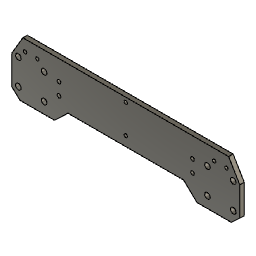
lcd_cover_prusa (Autodesk Fusion 360 archive; units mm, degrees)
design "front_plate"
Autodesk Fusion 360 part; units mm, degrees
sketch "MK3-front-plate" plane through (0, 0, 0) normal (0, 1, 0) x (1, 0, 0)
  line L0 (-64, 0) -> (-95, 0)
  line L1 (-95, 0) -> (-102.5, -7)
  line L2 (-102.5, -7) -> (-102.5, -33)
  line L3 (-102.5, -33) -> (-92.5, -50)
  line L4 (-92.5, -50) -> (92.5, -50)
  line L5 (102.5, -33) -> (102.5, -7)
  line L6 (64, 0) -> (52, -11.5)
  line L7 (102.5, -7) -> (95, 0)
  line L8 (-52, -11.5) -> (-64, 0)
  line L9 (95, 0) -> (64, 0)
  line L10 (52, -11.5) -> (-52, -11.5)
  line L11 (92.5, -50) -> (102.5, -33)
  line L12 (-64, 0) -> (64, 0) construction
  line L13 (-73.4, 0) -> (-73.4, -50) construction
  line L14 (-96.6, 0) -> (-96.6, -50) construction
  circle A0 centre (-73.4, -9.9) radius 2.5
  circle A1 centre (-96.6, -9.9) radius 2.5
  circle A2 centre (-73.4, -33.1) radius 2.5
  circle A3 centre (-96.6, -33.1) radius 2.5
  line L15 (-96.6, -40) -> (-73.4, -40) construction
  circle A4 centre (-90.5, -40) radius 1.5
  circle A5 centre (-79.5, -40) radius 1.5
  circle A6 centre (0, -46) radius 1.5
  line L16 (0, 0) -> (0, -50) construction
  circle A7 centre (0, -20) radius 1.5
  line L17 (-60, -21) -> (-60, -32) construction
  circle A8 centre (-60, -21) radius 1.65
  circle A9 centre (-60, -32) radius 1.65
  circle A10 centre (60, -32) radius 1.65
  circle A11 centre (60, -21) radius 1.65
  circle A12 centre (73.4, -9.9) radius 2.5
  circle A13 centre (96.6, -9.9) radius 2.5
  circle A14 centre (96.6, -33.1) radius 2.5
  circle A15 centre (73.4, -33.1) radius 2.5
  circle A16 centre (79.5, -40) radius 1.5
  circle A17 centre (90.5, -40) radius 1.5
  line L18 (0, -33.1) -> (-102.5, -33.1) construction
  line L19 (-102.5, -9.9) -> (0, -9.9) construction
  dimension "d3" = 50
  dimension "d4" = 205
  dimension "d5" = 7.5
  dimension "d12" = 10
  dimension "d16" = 17
  dimension "d26" = 5
  dimension "d27" = 5
  dimension "d28" = 5
  dimension "d29" = 5
  dimension "d37" = 3
  dimension "d40" = 3
  dimension "d46" = 4
  dimension "d48" = 3
  dimension "d49" = 3
  dimension "d50" = 10
  dimension "d51" = 16.9
  dimension "d52" = 3.3
  dimension "d53" = 3.3
  dimension "d54" = 18
  dimension "d56" = 42.5
  dimension "d57" = 5.9
  dimension "d58" = 29.1
  dimension "d59" = 40.1
  dimension "d60" = 102.5
  dimension "d61" = 43
  dimension "d62" = 29
  dimension "d63" = 12
  dimension "d64" = 23
  dimension "d65" = 50.5
  dimension "d66" = 12
  dimension "d67" = 38.5
  dimension "d68" = 30
  constraint parallel L9 L12
  constraint midpoint L16.start L12
  constraint coincident L0 L13.start
  constraint coincident L4 L13.end
  constraint perpendicular L4 L13
  constraint coincident L0 L14.start
  constraint coincident L4 L14.end
  constraint perpendicular L4 L14
  constraint coincident L2 L19.start
  constraint coincident L2 L18.end
  constraint coincident L13 A0.centre
  constraint coincident A0.centre L19
  constraint coincident L14 A1.centre
  constraint coincident A1.centre L19
  constraint coincident L13 A2.centre
  constraint coincident L14 A3.centre
  constraint coincident L14 L15.start
  constraint coincident L13 L15.end
  constraint perpendicular L13 L15
  constraint coincident L15 A4.centre
  constraint coincident L15 A5.centre
  constraint coincident L16.start origin
  constraint midpoint L4 L16.end
  constraint coincident L16 A7.centre
  constraint coincident A6.centre L16
  constraint symmetric L3 L11 L16
  constraint symmetric L1 L7 L16
  constraint coincident L17.start A8.centre
  constraint coincident L17.end A9.centre
  constraint vertical L17
  constraint symmetric L16 A8 A11
  constraint symmetric L16 A9 A10
  constraint symmetric L2 L5 L16
  constraint symmetric A0 L16 A12
  constraint symmetric A1 L16 A13
  constraint symmetric A2 L16 A15
  constraint symmetric A3 L16 A14
  constraint symmetric A4 L16 A17
  constraint symmetric A5 L16 A16
  constraint symmetric L6 L8 L16
  constraint coincident L16 L18.start
  constraint coincident L16 L19.end
  constraint perpendicular L16 L18
  constraint perpendicular L16 L19
  constraint coincident A2.centre L18
  constraint coincident A3.centre L18
  measures "d3" distance of L0 L4
  measures "d4" distance of L2 L5
  measures "d5" distance of L0.end L2
  measures "d12" horizontal distance of L2.end L3.end
  measures "d16" vertical distance of L2.end L3.end
  measures "d26" diameter of A0
  measures "d27" diameter of A1
  measures "d28" diameter of A2
  measures "d29" diameter of A3
  measures "d37" diameter of A4
  measures "d40" diameter of A5
  measures "d46" distance of L4 A6.centre
  measures "d48" diameter of A7
  measures "d49" diameter of A6
  measures "d50" distance of L4 L15.end
  measures "d51" vertical distance of L3.end L18.end
  measures "d52" diameter of A9
  measures "d53" diameter of A8
  measures "d54" distance of L4 L17.end
  measures "d56" distance of L2 L17.end
  measures "d57" horizontal distance of L1.end L14.start
  measures "d58" horizontal distance of L1.end L13.start
  measures "d59" vertical distance of L3.end L19.start
  measures "d60" horizontal distance of L16.start L1.end
  measures "d61" vertical distance of L1.end L3.end
  measures "d62" distance of L4 L17.start
  measures "d63" horizontal distance of L18.end A4.centre
  measures "d64" horizontal distance of L18.end A5.centre
  measures "d65" horizontal distance of L1.end L8.start
  measures "d66" horizontal distance of L0.start L8.start
  measures "d67" distance of L4 L10
  measures "d68" distance of L4 A7.centre
extrude "Extrude1" add sketch "MK3-front-plate" along normal blind 4
equation "d38 = ( ( 23.2 - 11 ) / 2 ) * 1 mm"
equation "d43 = ( ( 23.2 - 11 ) / 2 ) * 1 mm"

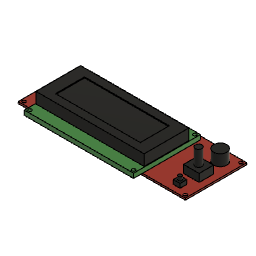
design "lcd"
Autodesk Fusion 360 part; units mm, degrees
sketch "Sketch1" plane through (0, 0, 0) normal (0, 0, 1) x (1, 0, 0)
  line L0 (150, 55) -> (150, 0)
  line L1 (150, 0) -> (0, 0)
  line L2 (0, 55) -> (150, 55)
  line L3 (68.5, 32.5) -> (66.3, 32.5) construction
  line L4 (66.3, 32.5) -> (66.3, 23.5)
  line L5 (0, 0) -> (0, 55)
  line L6 (89, 32.5) -> (89, 23.5)
  line L7 (45.8, 32.5) -> (66.3, 32.5)
  line L8 (89, 23.5) -> (68.5, 23.5)
  line L9 (66.3, 23.5) -> (45.8, 23.5)
  line L10 (68.5, 32.5) -> (89, 32.5)
  line L11 (68.5, 23.5) -> (68.5, 32.5)
  line L12 (45.8, 23.5) -> (45.8, 32.5)
  circle A0 centre (2.6, 2.6) radius 1.5
  circle A1 centre (2.6, 52.4) radius 1.5
  circle A2 centre (147.4, 52.4) radius 1.5
  circle A3 centre (147.4, 2.6) radius 1.5
  line L13 (2.6, 52.4) -> (147.4, 52.4) construction
  line L14 (147.4, 52.4) -> (147.4, 2.6) construction
  line L15 (147.4, 2.6) -> (2.6, 2.6) construction
  line L16 (2.6, 2.6) -> (2.6, 52.4) construction
  line L17 (13.5, 52) -> (111.5, 52)
  line L18 (111.5, 52) -> (111.5, -8)
  line L19 (111.5, -8) -> (13.5, -8)
  line L20 (13.5, -8) -> (13.5, 52)
  line L21 (13.5, 42) -> (111.5, 42)
  line L22 (13.5, 2) -> (111.5, 2)
  line L23 (75, 52.4) -> (75, 55) construction
  line L24 (14, 42) -> (14, 2)
  line L25 (111, 42) -> (111, 2)
  circle A4 centre (137, 44.2) radius 6
  line L26 (137, 44.2) -> (137, 8.2) construction
  line L27 (130, 31.3) -> (144, 31.3)
  line L28 (144, 31.3) -> (144, 18.3)
  line L29 (144, 18.3) -> (130, 18.3)
  line L30 (130, 18.3) -> (130, 31.3)
  line L31 (130, 24.8) -> (144, 24.8) construction
  line L32 (134, 11.2) -> (140, 11.2)
  line L33 (140, 11.2) -> (140, 5.2)
  line L34 (140, 5.2) -> (134, 5.2)
  line L35 (134, 5.2) -> (134, 11.2)
  line L36 (140, 8.2) -> (134, 8.2) construction
  circle A5 centre (137, 24.8) radius 3
  line L37 (0, 27.5) -> (150, 27.5) construction
  circle A6 centre (137, 8.2) radius 1.6
  line L38 (0, 8.5) -> (26.5, 8.5)
  line L39 (26.5, 8.5) -> (26.5, 35)
  line L40 (26.5, 35) -> (0, 35)
  line L41 (1, 8.5) -> (1, 35)
  circle A7 centre (16, -5.5) radius 1.5
  circle A8 centre (16, 49.5) radius 1.5
  circle A9 centre (109, -5.5) radius 1.5
  circle A10 centre (109, 49.5) radius 1.5
  line L42 (16, 49.5) -> (16, -5.5) construction
  line L43 (109, 49.5) -> (109, -5.5) construction
  line L44 (109, 49.5) -> (16, 49.5) construction
  line L45 (16, -5.5) -> (109, -5.5) construction
  point P0 (2.6, 27.5)
  dimension "d64" = 9
  dimension "d65" = 9
  dimension "d66" = 20.5
  dimension "d67" = 20.5
  dimension "d70" = 61
  dimension "d71" = 55
  dimension "d72" = 150
  dimension "d77" = 3
  dimension "d78" = 3
  dimension "d79" = 3
  dimension "d80" = 3
  dimension "d83" = 144.8
  dimension "d84" = 49.8
  dimension "d87" = 60
  dimension "d88" = 98
  dimension "d90" = 13.5
  dimension "d91" = 40
  dimension "d94" = 10
  dimension "d108" = 13
  dimension "d111" = 13
  dimension "d112" = 14
  dimension "d113" = 12
  dimension "d114" = 6
  dimension "d115" = 6
  dimension "d116" = 6
  dimension "d1" = 10.6
  dimension "d2" = 2.7
  dimension "d4" = 22.5
  dimension "d5" = 43.2
  dimension "d6" = 19.3
  dimension "d7" = 3.2
  dimension "d12" = 16.7
  dimension "d13" = 26.5
  dimension "d14" = 26.5
  dimension "d19" = 1
  dimension "d20" = 7.5
  dimension "d27" = 3
  dimension "d28" = 3
  dimension "d29" = 3
  dimension "d30" = 3
  dimension "d31" = 93
  dimension "d32" = 2.5
  dimension "d33" = 55
  dimension "d34" = 2.5
  dimension "d36" = 0.5
  dimension "d37" = 0.5
  constraint horizontal L2
  constraint vertical L0
  constraint horizontal L1
  constraint vertical L5
  constraint horizontal L8
  constraint vertical L11
  constraint horizontal L10
  constraint vertical L6
  constraint horizontal L9
  constraint vertical L12
  constraint horizontal L7
  constraint vertical L4
  constraint perpendicular L3 L11
  constraint coincident L1.end L5.start
  constraint horizontal L13
  constraint vertical L14
  constraint horizontal L15
  constraint vertical L16
  constraint coincident A1.centre L13.start
  constraint coincident A0.centre L15.end
  constraint coincident A3.centre L14.end
  constraint coincident A2.centre L13.end
  constraint horizontal L17
  constraint vertical L18
  constraint horizontal L19
  constraint vertical L20
  constraint coincident L20 L21.start
  constraint coincident L18 L21.end
  constraint perpendicular L18 L21
  constraint coincident L20 L22.start
  constraint coincident L18 L22.end
  constraint perpendicular L20 L22
  constraint midpoint L13 L23.start
  constraint midpoint L2 L23.end
  constraint perpendicular L2 L23
  constraint coincident L21 L24.start
  constraint coincident L22 L24.end
  constraint perpendicular L22 L24
  constraint coincident L21 L25.start
  constraint coincident L22 L25.end
  constraint perpendicular L22 L25
  constraint coincident A4.centre L26.start
  constraint vertical L26
  constraint horizontal L27
  constraint vertical L28
  constraint horizontal L29
  constraint vertical L30
  constraint midpoint L30 L31.start
  constraint midpoint L28 L31.end
  constraint symmetric L26 L28 L30
  constraint horizontal L32
  constraint vertical L33
  constraint horizontal L34
  constraint vertical L35
  constraint midpoint L33 L36.start
  constraint midpoint L35 L36.end
  constraint midpoint L26.end L36
  constraint midpoint L31 A5.centre
  constraint midpoint L5 L37.start
  constraint midpoint L0 L37.end
  constraint coincident L16 P0
  constraint midpoint L16 P0
  constraint coincident L37 P0
  constraint coincident L26.end A6.centre
  constraint coincident L5 L38.start
  constraint perpendicular L16 L38
  constraint perpendicular L38 L39
  constraint coincident L5 L40.end
  constraint perpendicular L5 L40
  constraint coincident L38 L41.start
  constraint coincident L40 L41.end
  constraint perpendicular L40 L41
  constraint coincident A8.centre L42.start
  constraint coincident A7.centre L42.end
  constraint vertical L42
  constraint coincident A10.centre L43.start
  constraint coincident A9.centre L43.end
  constraint vertical L43
  constraint horizontal L44
  constraint horizontal L45
  measures "d64" vertical distance of L6.start L6.end
  measures "d65" vertical distance of L7.start L9.end
  measures "d66" horizontal distance of L6.end L8.end
  measures "d67" horizontal distance of L4.end L9.end
  measures "d70" horizontal distance of L6.start L0.start
  measures "d71" distance of L2.start L1.end
  measures "d72" distance of L0.start L2.start
  measures "d77" diameter of A1
  measures "d78" diameter of A2
  measures "d79" diameter of A3
  measures "d80" diameter of A0
  measures "d83" distance of A1.centre A2.centre
  measures "d84" distance of A0.centre A1.centre
  measures "d87" distance of L17.start L19.end
  measures "d88" distance of L17.start L17.end
  measures "d90" horizontal distance of L2.start L17.start
  measures "d91" distance of L21.end L22.end
  measures "d94" distance of L17.end L21.end
  measures "d108" horizontal distance of L0.end L26.end
  measures "d111" distance of L27.end L28.end
  measures "d112" distance of L27.start L27.end
  measures "d113" diameter of A4
  measures "d114" distance of L32.end L33.end
  measures "d115" distance of L32.start L32.end
  measures "d116" diameter of A5
  measures "d1" vertical distance of A0.centre L19.end
  measures "d2" vertical distance of L31.end L37.end
  measures "d4" distance of L2 L10
  measures "d5" distance of L6 L12
  measures "d6" vertical distance of L36.start L37.end
  measures "d7" diameter of A6
  measures "d12" vertical distance of A4.centre L37.end
  measures "d13" distance of L38 L40
  measures "d14" distance of L38.start L38.end
  measures "d19" distance of L5 L41
  measures "d20" distance of L37.start L40
  measures "d27" diameter of A7
  measures "d28" diameter of A9
  measures "d29" diameter of A10
  measures "d30" diameter of A8
  measures "d31" horizontal distance of A7.centre A9.centre
  measures "d32" distance of L18 A9.centre
  measures "d33" vertical distance of A7.centre A8.centre
  measures "d34" distance of L19 A7.centre
  measures "d36" distance of L20 L24
  measures "d37" distance of L18 L25
extrude "Extrude1" add sketch "Sketch1" along normal blind 1.6 contours L0 L1 L2 L5 L17 L18 L20 L40 | L1 L18 L20 L22 | L5 L38 L40 L41 | L1 L5 L20 L38 | L18 L21 L22 L25 | L20 L38 L40 L41 | L20 L22 L24 L38 | L17 L18 L20 L21 | L21 L22 L24 L25 L38 L39 L40 | L20 L24 L38 L40 | L20 L21 L24 L40 | L24 L38 L39 L40 | L4 L7 L9 L12 | L6 L8 L10 L11 | A4 | L27 L28 L29 L30 | L32 L33 L34 L35 | A5 | A6 | A8 | A10
extrude "Extrude2" add sketch "Sketch1" against normal blind 9 contours L4 L7 L9 L12 | L6 L8 L10 L11
extrude "Extrude3" add sketch "Sketch1" along normal blind 4.1 from surface at 1.6 contours L1 L18 L19 L20 | L1 L18 L20 L22 | L18 L21 L22 L25 | L20 L22 L24 L38 | L17 L18 L20 L21 | L21 L22 L24 L25 L38 L39 L40 | L20 L24 L38 L40 | L20 L21 L24 L40 | L24 L38 L39 L40 | L4 L7 L9 L12 | L6 L8 L10 L11
extrude "Extrude4" add sketch "Sketch1" along normal blind 9.8 from surface at 5.7 contours L21 L22 L24 L25 L38 L39 L40 | L24 L38 L39 L40 | L4 L7 L9 L12 | L6 L8 L10 L11
extrude "Extrude5" add sketch "Sketch1" along normal blind 10 from surface at 1.6 contours A4
extrude "Extrude6" add sketch "Sketch1" along normal blind 7 from surface at 1.6 contours L27 L28 L29 L30 | A5
extrude "Extrude7" add sketch "Sketch1" along normal blind 14 from surface at 8.6 contours A5
extrude "Extrude8" add sketch "Sketch1" along normal blind 3.8 from surface at 1.6 contours L32 L33 L34 L35 | A6
extrude "Extrude9" add sketch "Sketch1" along normal blind 7 from surface at 1.6 contours A6
extrude "Extrude10" add sketch "Sketch1" against normal blind 3 contours L20 L38 L40 L41 | L20 L24 L38 L40 | L24 L38 L39 L40
sketch "Sketch2" plane through (0, 0, 15.5) normal (0, 0, 1) x (-1, 0, 0)
  line L0 (-111, -42) -> (-14, -42)
  line L1 (-14, -42) -> (-14, -2)
  line L2 (-14, -2) -> (-111, -2)
  line L3 (-111, -2) -> (-111, -42)
  line L4 (-24.5, -35) -> (-100.5, -35)
  line L5 (-100.5, -35) -> (-100.5, -9)
  line L6 (-100.5, -9) -> (-24.5, -9)
  line L7 (-24.5, -9) -> (-24.5, -35)
  line L8 (-62.5, -42) -> (-62.5, -2) construction
  line L9 (-111, -22) -> (-14, -22) construction
  dimension "d23" = 76
  dimension "d24" = 26
  constraint horizontal L4
  constraint vertical L5
  constraint horizontal L6
  constraint vertical L7
  constraint midpoint L0 L8.start
  constraint midpoint L2 L8.end
  constraint midpoint L3 L9.start
  constraint midpoint L1 L9.end
  constraint symmetric L4 L6 L9
  measures "d23" distance of L5 L7
  measures "d24" distance of L4 L6
extrude "Extrude11" cut sketch "Sketch2" against normal blind 0.8 contours L4 L5 L6 L7
equation "d64 = d65"
equation "d78 = d77"
equation "d79 = d77"
equation "d80 = d77"
equation "d94 = ( d87 - d91 ) / 2"
equation "d28 = d27"
equation "d29 = d27"
equation "d30 = d27"
equation "d32 = ( d88 - d31 ) / 2"
equation "d34 = ( d87 - d33 ) / 2"
equation "d37 = d36"

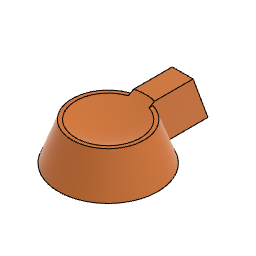
design "lcd_knob"
Autodesk Fusion 360 part; units mm, degrees
sketch "Sketch3" plane through (0, 0, 0) normal (1, 0, 0) x (0, 1, 0)
  line L0 (0, 0) -> (18, 0)
  line L1 (10, 0) -> (7.0154, 8.2)
  line L2 (0, 20) -> (0, 0)
  line L3 (0, 8.2) -> (15.0154, 8.2)
  arc A0 (0, 6) -> (7.5339, 8.2) centre (0, 20) ccw
  line L4 (18, 0) -> (15.0154, 8.2)
  dimension "d22" = 20
  dimension "d23" = 14
  dimension "d24" = 10
  dimension "d31" = 8
  dimension "d1" = 70
  dimension "d9" = 8.2
  constraint coincident L0.start L2.end
  constraint horizontal L0
  constraint perpendicular L0 L2
  constraint parallel L0 L3
  constraint coincident L2.start A0.centre
  constraint coincident L1.start L0
  constraint parallel L1 L4
  constraint coincident L3 L1.end
  constraint coincident A0.end L3
  constraint coincident L2 A0.start
  constraint coincident L2 L3.start
  measures "d22" distance of L0.start L2.start
  measures "d23" radius of A0
  measures "d24" distance of L0.start L1.start
  measures "d31" distance of L1.start L0.end
  measures "d1" angle of L0 L1
  measures "d9" distance of L0 L3
revolve "Revolve1" add sketch "Sketch3" angle 360 about axis through (0, 0, 20) along (0, 0, -1) contours L0 L1 L2 A0 | L1 L2 L3 A0
extrude "Extrude1" add sketch "Sketch3" along normal mid plane 4.2
revolve "Revolve2" cut sketch "Sketch3" angle 360 about axis through (0, 0, 20) along (0, 0, -1) contours L1 L2 L3 A0 | L1 L3 A0
sketch "Sketch4" plane through (0, 0, 8.2) normal (0, 0, 1) x (-1, 0, 0)
  line L0 (-2.1, -7.2353) -> (-2.1, -15.0154)
  line L1 (-2.1, -15.0154) -> (2.1, -15.0154)
  line L2 (2.1, -15.0154) -> (2.1, -7.2353)
  line L3 (2.1, -7.2353) -> (2.1, -5.2353)
  line L4 (2.1, -5.2353) -> (-2.1, -5.2353)
  line L5 (-2.1, -7.2353) -> (-2.1, -5.2353)
  circle A0 centre (0, 0) radius 9.0154
  line L6 (2.1, -7.2353) -> (2.1, -15.0154)
  line L7 (-2.1, -15.0154) -> (-2.1, -7.2353)
  dimension "d13" = 2
  constraint coincident L2.end L3.start
  constraint parallel L2 L3
  constraint perpendicular L3 L4
  constraint parallel L0 L5
  constraint coincident L0.start L5.start
  measures "d13" distance of L2.end L3.end
extrude "Extrude3" cut sketch "Sketch4" against normal blind 0.6 contours L0 L2 L3 L4 L5 A0 L6 L7 picked at (-0.2128, -0.4926)
sketch "Sketch1" plane through (0, 0, 0) normal (0, 0, -1) x (1, 0, 0)
  circle A0 centre (0, 0) radius 3
  circle A1 centre (0, 0) radius 5
  circle A2 centre (0, 0) radius 5.5
  line L0 (4.9749, -0.5) -> (2.958, -0.5)
  line L1 (4.9749, 0.5) -> (2.958, 0.5)
  line L2 (5, 0) -> (0, 0) construction
  line L3 (-2.1, -9.777) -> (-2.1, -18)
  line L4 (-2.1, -18) -> (2.1, -18)
  line L5 (2.1, -18) -> (2.1, -9.777)
  arc A3 (2.1, -9.777) -> (-2.1, -9.777) centre (0, 0) ccw
  dimension "d4" = 6
  dimension "d6" = 0.5
  dimension "d7" = 1
  dimension "d14" = 2
  constraint coincident A0.centre A1.centre
  constraint coincident A1 L0.start
  constraint coincident A0 L0.end
  constraint horizontal L0
  constraint coincident A1 L1.start
  constraint coincident A0 L1.end
  constraint parallel L0 L1
  constraint coincident A1 L2.start
  constraint horizontal L2
  constraint symmetric L0 L1 L2
  constraint concentric A2 A3
  measures "d4" diameter of A0
  measures "d6" distance of A1 A2
  measures "d7" distance of L0.start L1.start
  measures "d14" distance of A0 A1
extrude "Extrude2" cut sketch "Sketch1" against normal blind 4.6 contours A0 | A0 A1 L0 L1 | A2 picked at (3.6642, -0.1114)
chamfer "Chamfer1" distance 0.4 distance2 0.5 1 edges at (-3, 0, 0) measured on face at (-4.3242, 0, 0)
chamfer "Chamfer2" distance 0.225 distance2 0.9 2 edges at (-5, 0, 0) (-5.1278, -1.9889, 0) measured on face at (-4.4575, 0, 0) measured on face at (0.7, 12.518, 0)
